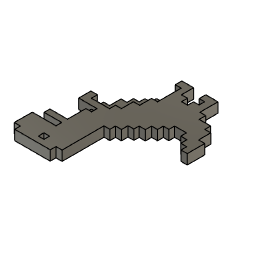
Dino_Keychain (Autodesk Fusion 360 design; units mm, degrees)
Autodesk Fusion 360 part; units mm, degrees
sketch "dino" plane through (0, 0, 0) normal (0, 0, 1) x (1, 0, 0)
  line L0 (-1, -5) -> (-41, -5)
  line L1 (-41, -5) -> (-41, 35)
  line L2 (-41, 35) -> (-1, 35)
  line L3 (-1, 35) -> (-1, -5)
  line L4 (-37.8669, -1.9758) -> (-36, -1.9758)
  line L5 (-36, -1.9758) -> (-36, -3.7206)
  line L6 (-36, -3.7206) -> (-25.1685, -3.7206)
  line L7 (-25.1685, -3.7206) -> (-25.1685, -1.9758)
  line L8 (-25.1685, -1.9758) -> (-23.3, -1.9758)
  line L9 (-23.3, -1.9758) -> (-23.3, 10.7954)
  line L10 (-23.3, 10.7954) -> (-21.5, 10.7954)
  line L11 (-21.5, 10.7954) -> (-21.5, 12.5)
  line L12 (-21.5, 12.5) -> (-19.672, 12.5)
  line L13 (-19.672, 12.5) -> (-19.672, 14.5)
  line L14 (-19.672, 14.5) -> (-17.9, 14.5)
  line L15 (-17.9, 14.5) -> (-17.9, 16.1)
  line L16 (-17.9, 16.1) -> (-16, 16.1)
  line L17 (-16, 16.1) -> (-16, 18)
  line L18 (-16, 18) -> (-14.189, 18)
  line L19 (-14.189, 18) -> (-14.189, 19.764)
  line L20 (-14.189, 19.764) -> (-12.5, 19.764)
  line L21 (-12.5, 19.764) -> (-12.5, 21.5)
  line L22 (-12.5, 21.5) -> (-8.8798, 21.5)
  line L23 (-8.8798, 21.5) -> (-8.8798, 19.764)
  line L24 (-8.8798, 19.764) -> (-7, 19.764)
  line L25 (-7, 19.764) -> (-7, 17.9)
  line L26 (-7, 17.9) -> (-5.1831, 17.9)
  line L27 (-5.1831, 17.9) -> (-5.1831, 16.1484)
  line L28 (-5.1831, 16.1484) -> (-3.2862, 16.1484)
  line L29 (-3.2862, 16.1484) -> (-3.2862, 21.5)
  line L30 (-3.2862, 21.5) -> (-5.1831, 21.5)
  line L31 (-5.1831, 21.5) -> (-5.1831, 25.233)
  line L32 (-5.1831, 25.233) -> (-7, 25.233)
  line L33 (-7, 25.233) -> (-7, 27)
  line L34 (-7, 27) -> (-10.5, 27)
  line L35 (-10.5, 27) -> (-10.5, 29)
  line L36 (-10.5, 29) -> (-12.276, 29)
  line L37 (-12.276, 29) -> (-12.276, 34.5)
  line L38 (-12.276, 34.5) -> (-16, 34.5)
  line L39 (-16, 34.5) -> (-16, 32.5)
  line L40 (-16, 32.5) -> (-14.3257, 32.5)
  line L41 (-14.3257, 32.5) -> (-14.3257, 30.7993)
  line L42 (-14.3257, 30.7993) -> (-16, 30.7993)
  line L43 (-16, 30.7993) -> (-16, 29)
  line L44 (-16, 29) -> (-17.8539, 29)
  line L45 (-17.8539, 29) -> (-17.8539, 30.7993)
  line L46 (-17.8539, 30.7993) -> (-19.6941, 30.7993)
  line L47 (-19.6941, 30.7993) -> (-19.6941, 34.5)
  line L48 (-19.6941, 34.5) -> (-23.2983, 34.5)
  line L49 (-23.2983, 34.5) -> (-23.2983, 32.5)
  line L50 (-23.2983, 32.5) -> (-21.4962, 32.5)
  line L51 (-21.4962, 32.5) -> (-21.4962, 25.308)
  line L52 (-21.4962, 25.308) -> (-23.2983, 25.308)
  line L53 (-23.2983, 25.308) -> (-23.2983, 21.6664)
  line L54 (-23.2983, 21.6664) -> (-25.1992, 21.6664)
  line L55 (-25.1992, 21.6664) -> (-25.1992, 18)
  line L56 (-25.1992, 18) -> (-27, 18)
  line L57 (-27, 18) -> (-27, 16.1853)
  line L58 (-27, 16.1853) -> (-30.633, 16.1853)
  line L59 (-30.633, 16.1853) -> (-30.633, 7)
  line L60 (-30.633, 7) -> (-36, 7)
  line L61 (-36, 7) -> (-36, 5.2364)
  line L62 (-36, 5.2364) -> (-30.633, 5.2364)
  line L63 (-30.633, 5.2364) -> (-30.633, 3.5)
  line L64 (-30.633, 3.5) -> (-37.8295, 3.5)
  line L65 (-37.8295, 3.5) -> (-37.8669, -1.9758)
  line L66 (-30.6, -1.9) -> (-28.9, -1.9)
  line L67 (-28.9, -1.9) -> (-28.9, -0.2)
  line L68 (-28.9, -0.2) -> (-30.633, -0.2)
  line L69 (-30.633, -0.2) -> (-30.6, -1.9)
  line L70 (-30.633, 12.6033) -> (-28.9, 12.6033)
  line L71 (-28.9, 12.6033) -> (-28.9, 14.2784)
  line L72 (-28.9, 14.2784) -> (-34.5, 14.2784)
  line L73 (-34.5, 14.2784) -> (-34.5, 18)
  line L74 (-34.5, 18) -> (-32.5, 18)
  line L75 (-32.5, 18) -> (-32.5, 16.1392)
  line L76 (-32.5, 16.1392) -> (-30.633, 16.1853)
  line L77 (-30.633, 17.9928) -> (-28.8165, 17.9928)
  line L78 (-28.8165, 17.9928) -> (-28.8165, 21.5)
  line L79 (-28.8165, 21.5) -> (-27, 21.5)
  line L80 (-27, 21.5) -> (-27, 23.5)
  line L81 (-27, 23.5) -> (-25.274, 23.5)
  line L82 (-25.274, 23.5) -> (-25.274, 25.1824)
  line L83 (-25.274, 25.1824) -> (-23.5, 25.1824)
  line L84 (-23.5, 25.1824) -> (-23.5, 27)
  line L85 (-23.5, 27) -> (-21.4962, 27)
  line L86 (-30.633, 17.9928) -> (-30.633, 16.1853)
  dimension "d1" = 40
  dimension "d2" = 40
  constraint horizontal L0
  constraint vertical L1
  constraint horizontal L2
  constraint vertical L3
  constraint horizontal L4
  constraint perpendicular L4 L5
  constraint perpendicular L5 L6
  constraint perpendicular L6 L7
  constraint perpendicular L7 L8
  constraint perpendicular L8 L9
  constraint perpendicular L9 L10
  constraint perpendicular L10 L11
  constraint perpendicular L9 L12
  constraint perpendicular L0 L13
  constraint perpendicular L13 L14
  constraint perpendicular L14 L15
  constraint perpendicular L13 L16
  constraint perpendicular L16 L17
  constraint perpendicular L17 L18
  constraint perpendicular L16 L19
  constraint perpendicular L17 L20
  constraint perpendicular L16 L21
  constraint perpendicular L21 L22
  constraint perpendicular L22 L23
  constraint perpendicular L21 L24
  constraint perpendicular L22 L25
  constraint perpendicular L17 L26
  constraint perpendicular L26 L27
  constraint perpendicular L27 L28
  constraint perpendicular L28 L29
  constraint perpendicular L29 L30
  constraint perpendicular L18 L31
  constraint perpendicular L31 L32
  constraint perpendicular L18 L33
  constraint perpendicular L31 L34
  constraint perpendicular L18 L35
  constraint perpendicular L31 L36
  constraint perpendicular L2 L37
  constraint perpendicular L31 L38
  constraint perpendicular L38 L39
  constraint perpendicular L39 L40
  constraint perpendicular L40 L41
  constraint perpendicular L41 L42
  constraint perpendicular L42 L43
  constraint perpendicular L41 L44
  constraint perpendicular L44 L45
  constraint perpendicular L45 L46
  constraint perpendicular L46 L47
  constraint perpendicular L47 L48
  constraint perpendicular L48 L49
  constraint perpendicular L49 L50
  constraint perpendicular L2 L51
  constraint perpendicular L51 L52
  constraint perpendicular L2 L53
  constraint perpendicular L53 L54
  constraint perpendicular L54 L55
  constraint perpendicular L55 L56
  constraint perpendicular L56 L57
  constraint perpendicular L57 L58
  constraint perpendicular L58 L59
  constraint perpendicular L1 L60
  constraint perpendicular L60 L61
  constraint perpendicular L61 L62
  constraint perpendicular L62 L63
  constraint perpendicular L1 L64
  constraint perpendicular L59 L66
  constraint perpendicular L62 L67
  constraint perpendicular L59 L68
  constraint perpendicular L59 L70
  constraint perpendicular L70 L71
  constraint perpendicular L59 L72
  constraint perpendicular L72 L73
  constraint perpendicular L73 L74
  constraint perpendicular L74 L75
  constraint perpendicular L59 L77
  constraint perpendicular L77 L78
  constraint perpendicular L59 L79
  constraint perpendicular L77 L80
  constraint perpendicular L80 L81
  constraint perpendicular L81 L82
  constraint perpendicular L80 L83
  constraint perpendicular L83 L84
  constraint coincident L51 L85.end
  constraint perpendicular L51 L85
  constraint perpendicular L58 L86
  measures "d1" distance of L0.start L0.end
  measures "d2" distance of L0.start L2.end
extrude "Extrude1" add sketch "dino" along normal blind 3 contours L4 L5 L6 L7 L8 L9 L10 L11 L12 L13 L14 L15 L16 L17 L18 L19 L20 L21 L22 L23 L24 L25 L26 L27 L28 L29 L30 L31 L32 L33 L34 L35 L36 L37 L38 L39 L40 L41 L42 L43 L44 L45 L46 L47 L48 L49 L50 L51 L52 L53 L54 L55 L56 L57 L58 L59 L60 L61 L62 L63 L64 L65 L70 L71 L72 | L59 L72 L73 L74 L75 L76
extrude "Extrude2" add sketch "dino" along normal blind 2 and the other way blind -1 contours L59 L70 L71 L72 | L51 L52 L53 L54 L55 L56 L57 L58 L77 L78 L79 L80 L81 L82 L83 L84 L85 L86
named bodies: "dino"
